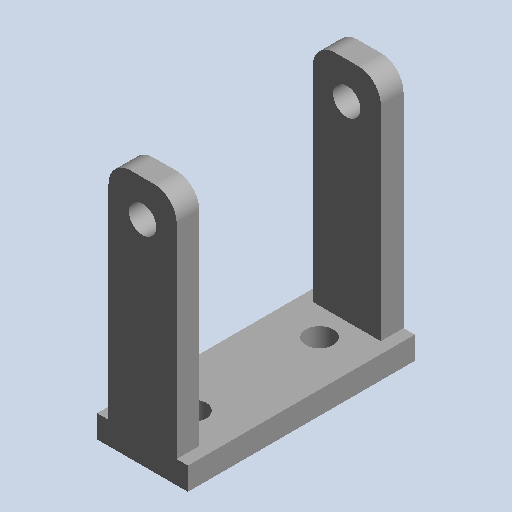
# Autodesk Inventor part: sensor_cover_ultrasonic_3
Saved by Autodesk Inventor 2026 (Build 300175050, 175E)
## iProperties
Part Number: sensor_cover_ultrasonic_3
Material: Generic
Document SubType Name: Modeling
Designer: Kartik
Mass: 11.8272 g
Surface Area: 67.6496 cm^2
Volume: 11.8272 cm^3
Density: 1 g/cm^3
Appearance: Default
Author: Kartik
Autodesk Inventor part; units mm, degrees
ref_plane "YZ Plane" through (0, 0, 0) normal (1, 0, 0) x (0, 1, 0)
ref_plane "XZ Plane" through (0, 0, 0) normal (0, 1, 0) x (-1, 0, 0)
ref_plane "XY Plane" through (0, 0, 0) normal (0, 0, 1) x (1, 0, 0)
sketch "Sketch1" plane through (0, 0, 0) normal (0, 1, 0) x (-1, 0, 0)
  line L0 (10, 25) -> (-10, 25)
  line L1 (-10, 25) -> (-10, -25)
  line L2 (-10, -25) -> (10, -25)
  line L3 (10, -25) -> (10, 25)
  point P0 (0, 0)
  dimension "d0" = 50
  dimension "d1" = 20
  dimension "d2" = 25
  dimension "d3" = 10
  constraints: 8 end point, 2 parallel, 1 horizontal, 1 perpendicular
  measures "d0" distance of L2.end L0.start
  measures "d1" distance of L0.start L0.end
  measures "d2" distance from line of L0 point (0, 0)
  measures "d3" distance from line of L3 point (0, 0)
extrude "Extrusion1" add sketch "Sketch1" along normal blind 5
sketch "Sketch2" plane through (0, 5, 0) normal (0, 1, 0) x (1, 0, 0)
  line L0 (-10, -25) -> (10, -25) projected
  line L1 (-7.5, -25) -> (7.5, -25)
  line L2 (7.5, -25) -> (7.5, -20)
  line L3 (7.5, -20) -> (-7.5, -20)
  line L4 (-7.5, -20) -> (-7.5, -25)
  line L5 (-10, 25) -> (-10, -25) projected
  line L6 (10, 25) -> (-10, 25) projected
  line L7 (-7.5, 25) -> (7.5, 25)
  line L8 (7.5, 25) -> (7.5, 20)
  line L9 (7.5, 20) -> (-7.5, 20)
  line L10 (-7.5, 20) -> (-7.5, 25)
  point P0 (0, 0)
  dimension "d6" = 15
  dimension "d7" = 5
  dimension "d8" = 2.5
  dimension "d9" = 5
  constraints: 16 end point, 4 parallel, 2 horizontal, 2 perpendicular, 2 point on line
  measures "d6" distance of L3.end L2.end
  measures "d7" distance of L2.end L1.end
  measures "d8" distance between parallel lines of L5 L4
  measures "d9" distance of L7.end L8.end
extrude "Extrusion2" add sketch "Sketch2" along normal blind 50
fillet "Fillet1" radius 5 4 edges at (7.5, 55, 22.5) (7.5, 55, -22.5) (-7.5, 55, 22.5) (-7.5, 55, -22.5)
sketch "Sketch3" plane through (-10, 0, 25) normal (0, 0, 1) x (1, 0, 0)
  line L0 (7.5, 55) -> (12.5, 55) projected
  circle A0 centre (10, 47) radius 3
  point P0 (10, 0)
  point P1 (10, 55)
  dimension "d13" = 6
  dimension "d14" = 8
  constraints: 1 centre point, 1 midpoint
  measures "d13" diameter of A0
  measures "d14" distance of point (10, 55) A0.centre
extrude "Extrusion3" cut sketch "Sketch3" against normal through all
sketch "Sketch4" plane through (0, 5, 0) normal (0, 1, 0) x (1, 0, 0)
  line L0 (2.5, -20) -> (-2.5, -20) projected
  line L1 (-2.5, 20) -> (2.5, 20) projected
  circle A0 centre (0, -14.0028) radius 3
  circle A1 centre (0, 14) radius 3
  point P0 (0, 0)
  point P1 (0, -20)
  dimension "d17" = 6
  dimension "d18" = 6
  dimension "d19" = 5.9972
  dimension "d20" = 6
  constraints: 2 centre point, 1 midpoint
  measures "d17" diameter of A0
  measures "d18" diameter of A1
  measures "d19" distance of point (0, -20) A0.centre
  measures "d20" distance from line of L1 A1.centre
extrude "Extrusion4" cut sketch "Sketch4" against normal blind 10
equation "\"d2\" = 0.5 * d0"
equation "\"d3\" = 0.5 * d1"
body "Solid1"
